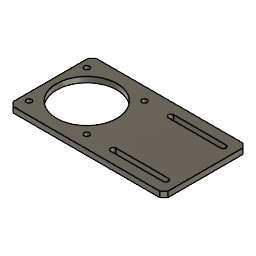
_Nema 34 Mounting Plate.8a0da9ef-3de6-49f1-ac7f-0628538dbad4 (Autodesk Fusion 360 design; units mm, degrees)
Autodesk Fusion 360 part; units mm, degrees
sketch "Sketch1" plane through (0, 0, 0) normal (0, 0, 1) x (1, 0, 0)
  line L0 (0, 0) -> (188, 0)
  line L1 (188, 0) -> (188, 101)
  line L2 (188, 101) -> (0, 101)
  line L3 (0, 101) -> (0, 0)
  circle A0 centre (44, 50.5) radius 36.5
  line L4 (0, 50.5) -> (188, 50.5) construction
  line L5 (9, 85.5) -> (79, 85.5) construction
  line L6 (79, 85.5) -> (79, 15.5) construction
  line L7 (79, 15.5) -> (9, 15.5) construction
  line L8 (9, 15.5) -> (9, 85.5) construction
  circle A1 centre (9, 85.5) radius 3.2
  circle A2 centre (79, 85.5) radius 3.2
  circle A3 centre (79, 15.5) radius 3.2
  circle A4 centre (9, 15.5) radius 3.2
  line L9 (111.2, 12.3) -> (174.8, 12.3)
  arc A5 (174.8, 12.3) -> (174.8, 18.7) centre (174.8, 15.5) ccw
  line L10 (174.8, 18.7) -> (111.2, 18.7)
  arc A6 (111.2, 18.7) -> (111.2, 12.3) centre (111.2, 15.5) ccw
  line L11 (111.2, 15.5) -> (174.8, 15.5) construction
  line L12 (111.2, 82.3) -> (174.8, 82.3)
  arc A7 (174.8, 82.3) -> (174.8, 88.7) centre (174.8, 85.5) ccw
  line L13 (174.8, 88.7) -> (111.2, 88.7)
  arc A8 (111.2, 88.7) -> (111.2, 82.3) centre (111.2, 85.5) ccw
  line L14 (111.2, 85.5) -> (174.8, 85.5) construction
  point P0 (44, 85.5)
  point P1 (9, 50.5)
  point P2 (178, 85.5)
  point P3 (108, 85.5)
  dimension "d1" = 188
  dimension "d2" = 101
  dimension "d3" = 73
  dimension "d4" = 70
  dimension "d5" = 6.4
  dimension "d6" = 9
  dimension "d7" = 10
  dimension "d8" = 70
  constraint horizontal L0
  constraint vertical L1
  constraint horizontal L2
  constraint vertical L3
  constraint coincident L0.start L3.end
  constraint midpoint L3 L4.start
  constraint midpoint L1 L4.end
  constraint coincident A0.centre L4
  constraint horizontal L5
  constraint vertical L6
  constraint horizontal L7
  constraint vertical L8
  constraint equal L5 L8
  constraint midpoint L5 P0
  constraint vertical A0.centre P0
  constraint midpoint L8 P1
  constraint horizontal A0.centre P1
  constraint coincident L5.start L8.end
  constraint coincident L5.end L6.start
  constraint coincident L6.end L7.start
  constraint coincident L7.end L8.start
  constraint equal A3 A4
  constraint equal A2 A3
  constraint equal A1 A2
  constraint tangent L9 A5
  constraint tangent A5 L10
  constraint parallel L9 L10
  constraint tangent L10 A6
  constraint tangent L9 A6
  constraint horizontal L11
  constraint tangent L12 A7
  constraint tangent A7 L13
  constraint parallel L12 L13
  constraint tangent L13 A8
  constraint tangent L12 A8
  constraint parallel L10 L14
  constraint equal A2 A7
  constraint equal A3 A5
  constraint coincident L6.end L11
  constraint coincident L5.end L14
  constraint equal L11 L14
  constraint midpoint A7 P2
  constraint vertical A5.centre A7.centre
  constraint midpoint A8 P3
  measures "d1" distance of L0.start L0.end
  measures "d2" distance of L0.start L2.end
  measures "d3" diameter of A0
  measures "d4" distance of L5.start L7.end
  measures "d5" diameter of A1
  measures "d6" distance of L3 L7.end
  measures "d7" distance of L1 P2
  measures "d8" distance of P2 P3
extrude "Extrude1" add sketch "Sketch1" along normal blind 6.8
chamfer "Chamfer1" distance 5 angle 45 4 edges at (188, 101, 3.4) (188, 0, 3.4) (0, 0, 3.4) (0, 101, 3.4)
